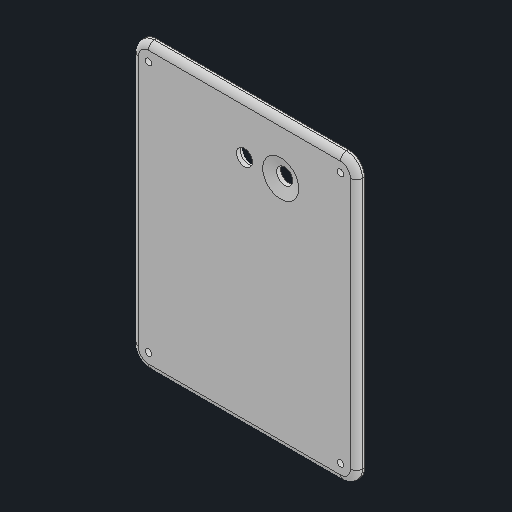
# Autodesk Inventor part: Lid
Saved by Autodesk Inventor 2026.2 (Build 302298000, 298)
## iProperties
Created: 2026-02-21
Part Number: Lid
Material: Generic
Document SubType Name: Modeling
Designer: niuke
Density: 1 g/cm^3
Appearance: Default
Author: niuke
Autodesk Inventor part; units mm, degrees
ref_plane "YZ Plane" through (0, 0, 0) normal (1, 0, 0) x (0, 1, 0)
sketch "Sketch1" plane through (0, 0, 0) normal (0, 0, 1) x (1, 0, 0)
  circle A0 centre (0, 0) radius 4 projected
  circle A1 centre (-18.1, 0) radius 2.9 construction
  circle A2 centre (29.9, -108.4) radius 1.6
  circle A3 centre (-66.1, -108.4) radius 1.6
  circle A4 centre (-66.1, 17.4) radius 1.6
  circle A5 centre (29.9, 17.4) radius 1.6
  line L0 (29.9, 17.4) -> (-66.1, 17.4) construction
  line L1 (37.9, -116.4) -> (-74.1, -116.4)
  line L2 (-74.1, -116.4) -> (-74.1, 25.4)
  line L3 (-74.1, 25.4) -> (37.9, 25.4)
  line L4 (37.9, 25.4) -> (37.9, -116.4)
  line L5 (-66.1, -108.4) -> (-66.1, 17.4) construction
  circle A6 centre (-18.1, 0) radius 4
  point P0 (-18.1, 17.4)
  point P1 (-18.1, 25.4)
  point P2 (-66.1, -45.5)
  point P3 (-74.1, -45.5)
  dimension "d0" = 3.2
  dimension "d1" = 96
  dimension "d2" = 125.8
  dimension "d3" = 141.8
  dimension "d4" = 112
  dimension "d5" = 25.4
  dimension "d11" = 8
  constraints: 12 end point, 5 centre point, 4 midpoint, 4 vertical alignment, 3 equal radius, 3 horizontal alignment, 2 horizontal, 2 parallel, 2 perpendicular, 1 coincident
  measures "d0" diameter of A2
  measures "d1" distance of L0.end L0.start
  measures "d2" distance of L0.start A2.centre
  measures "d3" distance of L3.end L1.start
  measures "d4" distance between parallel lines of L2 L4
  measures "d5" distance of point (-18.1, 25.4) A1.centre
  measures "d11" diameter of A6
ref_plane "Work Plane1" through (-18.1, 0, 3.4982) normal (0, 0, 1) x (1, 0, 0)
extrude "Extrusion1" add sketch "Sketch1" along normal blind 4
chamfer "Chamfer1" distance 5 distance2 2 1 edges at (-4, 0, 4) measured on face at (-17.9393, -72.8829, 4)
fillet "Fillet1" radius 8 4 edges at (37.9, 25.4, 2) (-74.1, 25.4, 2) (-74.1, -116.4, 2) (37.9, -116.4, 2)
sketch "Sketch2" plane through (0, 0, 4) normal (0, 0, 1) x (1, 0, 0)
  line L0 (32.7, -97.35) -> (-68.9, -97.35) construction
  line L1 (-68.9, -97.35) -> (-68.9, 4.25) construction
  line L2 (-68.9, 4.25) -> (32.7, 4.25) construction
  line L3 (32.7, 4.25) -> (32.7, -97.35) construction
  line L4 (-66.1, -116.4) -> (29.9, -116.4) construction
  point P0 (0, 0)
  point P1 (-18.1, -116.4)
  point P2 (-18.1, -97.35)
  dimension "d25" = 101.6
  dimension "d31" = 19.05
  constraints: 2 midpoint, 1 horizontal, 1 vertical alignment, 2 other
  measures "d25" distance of L0.start L0.end
  measures "d31" distance between parallel lines of L0 L4
fillet "Fillet2" radius 2 1 edges at (-22.1, 0, 0)
sketch "Sketch3" plane through (0, 0, 0) normal (0, 0, -1) x (-1, 0, 0)
  circle A0 centre (43.1, -6) radius 1 construction
  circle A1 centre (-8.9, 5) radius 1 construction
  circle A2 centre (43.1, -6) radius 0.75
  circle A3 centre (-8.9, 5) radius 0.75
  circle A4 centre (43.1, -6) radius 1.9
  circle A5 centre (-8.9, 5) radius 1.9
  point P0 (0, 0)
  dimension "d33" = 1.5
  dimension "d34" = 3.8
  constraints: 4 centre point, 4 coincident, 2 equal radius
  measures "d33" diameter of A2
  measures "d34" diameter of A4
ref_plane "Work Plane2" through (0, -10.5, -7.5) normal (0, 0, 1) x (1, 0, 0)
extrude "Extrusion2" add sketch "Sketch3" along normal up to surface (7.5 mm away)
fillet "Fillet3" radius 2 2 edges at (-41.2, -6, 0) (10.8, 5, 0)
fillet "Fillet4" radius 3 8 edges at (35.5569, 23.0569, 4) (-18.1, 25.4, 4) (-71.7569, 23.0569, 4) (-74.1, -45.5, 4) (-71.7569, -114.0569, 4) (-18.1, -116.4, 4) (35.5569, -114.0569, 4) (37.9, -45.5, 4)
body "Solid1"
